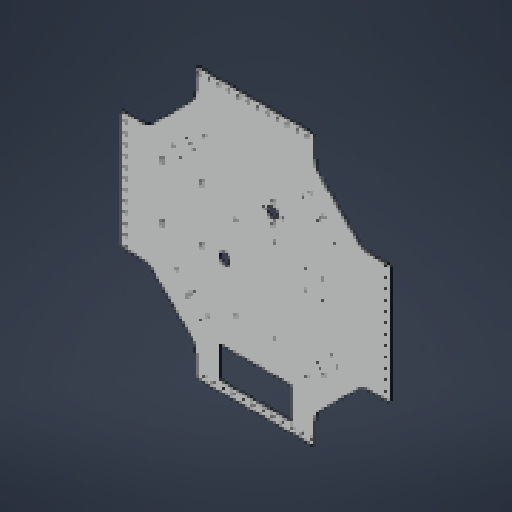
# Autodesk Inventor part: PLATE,MOUNT,ELECTRONICS
Saved by Autodesk Inventor 2026 (Build 300175000, 175)
## iProperties
Created: 2026-01-19
Part Number: PLATE,MOUNT,ELECTRONICS
Material: Aluminum 6061
Document SubType Name: Sheet Metal
Designer: Jthib
Mass: 2857.84 g
Surface Area: 7086.51 cm^2
Volume: 1058.46 cm^3
Density: 2.7 g/cm^3
Sheet Metal Rule: Default
Appearance: Aluminum - Flat
Flat Pattern Width: 69.85 cm
Flat Pattern Length: 69.85 cm
Flat Pattern Area: 4879.02 cm^2
Sheet Metal Width: 27.500 in
Sheet Metal Length: 27.500 in
Sheet Metal Area: 756.250 in^2
Author: Jthib
Autodesk Inventor part; units mm, degrees
ref_plane "YZ Plane" through (0, 0, 0) normal (1, 0, 0) x (0, 1, 0)
ref_plane "XZ Plane" through (0, 0, 0) normal (0, 1, 0) x (-1, 0, 0)
ref_plane "XY Plane" through (0, 0, 0) normal (0, 0, 1) x (1, 0, 0)
sketch "Sketch1" plane through (0, 0, 0) normal (0, 0, 1) x (1, 0, 0)
  line L0 (-298.45, -349.25) -> (298.45, -349.25)
  line L1 (349.25, -298.45) -> (349.25, 298.45)
  line L2 (298.45, 349.25) -> (-298.45, 349.25)
  line L3 (-349.25, 298.45) -> (-349.25, -298.45)
  line L4 (-349.25, -349.25) -> (349.25, 349.25) construction
  line L5 (349.25, -349.25) -> (-349.25, 349.25) construction
  arc A0 (349.25, 298.45) -> (298.45, 349.25) centre (298.45, 298.45) ccw
  arc A1 (-298.45, 349.25) -> (-349.25, 298.45) centre (-298.45, 298.45) ccw
  arc A2 (-349.25, -298.45) -> (-298.45, -349.25) centre (-298.45, -298.45) ccw
  arc A3 (298.45, -349.25) -> (349.25, -298.45) centre (298.45, -298.45) ccw
  point P0 (0, 0)
  dimension "d0" = 698.5
  dimension "d4" = 50.8
  measures "d0" distance of L4.end L5.end
  measures "d4" radius of A0
extrude "Plate1" add sketch "Sketch1" along normal blind 3.048
sketch "Sketch2" plane through (0, 0, 0) normal (0, 0, -1) x (-1, 0, 0)
  line L0 (-188.9125, -349.25) -> (-336.55, -349.25)
  arc A0 (-349.25, -336.55) -> (-336.55, -349.25) centre (-336.55, -336.55) ccw
  line L1 (-349.25, -336.55) -> (-349.25, -188.9125)
  line L2 (-153.035, -349.25) -> (-188.9125, -349.25)
  line L3 (-349.25, -188.9125) -> (-349.25, -153.035)
  line L4 (298.45, -349.25) -> (-298.45, -349.25) construction
  arc A1 (-270.7334, -168.4984) -> (-323.85, -190.5) centre (-292.735, -190.5) ccw construction
  line L5 (-270.7334, -168.4984) -> (-168.4984, -270.7334) construction
  arc A2 (-190.5, -323.85) -> (-168.4984, -270.7334) centre (-190.5, -292.735) ccw construction
  arc A3 (-266.2432, -164.0082) -> (-292.735, -153.035) centre (-292.735, -190.5) ccw
  line L6 (-266.2432, -164.0082) -> (-164.0082, -266.2432)
  arc A4 (-153.035, -292.735) -> (-164.0082, -266.2432) centre (-190.5, -292.735) ccw
  line L7 (-153.035, -349.25) -> (-153.035, -292.735)
  line L8 (-349.25, -153.035) -> (-292.735, -153.035)
  point P0 (0, 0)
  dimension "d10" = 6.35
  constraints: 16 end point, 10 point on circle, 5 centre point, 4 tangent, 2 perpendicular, 2 vertical, 1 collinear, 1 horizontal, 1 point on line, 15 other
  measures "d10" distance between parallel lines of L5 L6
extrude "Cut1" cut sketch "Sketch2" against normal blind 3.048
pattern_circular "Circular Pattern1" count 4 over 360 about axis through (0, 0, -10) along (0, 0, 1) of "Cut1"
fillet "Corner Round1" radius 6.35 8 edges at (-153.035, 349.25, 1.524) (349.25, -153.035, 1.524) (153.035, -349.25, 1.524) (-349.25, -153.035, 1.524) (-349.25, 153.035, 1.524) (-153.035, -349.25, 1.524) (153.035, 349.25, 1.524) (349.25, 153.035, 1.524)
sketch "Sketch3" plane through (0, 0, 0) normal (0, 0, -1) x (-1, 0, 0)
  line L0 (-146.685, 349.25) -> (146.685, 349.25) construction
  line L1 (-349.25, -146.685) -> (-349.25, 146.685) construction
  point P0 (0, 0)
  point P1 (-44.45, 120.65)
  point P2 (-19.05, 120.65)
  point P3 (-44.45, 146.05)
  point P4 (-69.85, 120.65)
  point P5 (-44.45, 95.25)
  dimension "d11" = 228.6
  dimension "d12" = 304.8
  dimension "d13" = 25.4
  dimension "d16" = 360
  constraints: 1 horizontal alignment, 5 other
  measures "d11" distance from line of L0 point (-44.45, 120.65)
  measures "d12" distance from line of L1 point (-44.45, 120.65)
  measures "d13" distance of point (-19.05, 120.65) point (-44.45, 120.65)
hole "Hole1" at (19.05, 120.65, 0) at (44.45, 146.05, 0) at (69.85, 120.65, 0) at (44.45, 95.25, 0) direction (0, 0, 1) diameter 5.1054 end through all clearance for "Flat Head Machine Screw (82)" size "#10" standard "Ansi Unified Screw Threads"
hole "Hole2" at (44.45, 120.65, 0) direction (0, 0, 1) diameter 28.575 end through all
sketch "Sketch4" plane through (0, 0, 3.048) normal (0, 0, 1) x (1, 0, 0)
  line L0 (-349.25, -146.685) -> (-349.25, 146.685) construction
  line L1 (-292.735, 153.035) -> (-342.9, 153.035) construction
  point P0 (0, 0)
  point P1 (-336.55, 133.35)
  dimension "d32" = 12.7
  dimension "d33" = 19.685
  measures "d32" distance from line of L0 point (-336.55, 133.35)
  measures "d33" distance from line of L1 point (-336.55, 133.35)
hole "Hole3" at (-336.55, 133.35, 3.048) direction (0, 0, -1) diameter 5.1054 end through all start extended yes clearance for "Flat Head Machine Screw (82)" size "#10" standard "Ansi Unified Screw Threads"
pattern_linear "Rectangular Pattern1" count 12 spacing 25.4 along (0, -1, 0) of "Hole3"
pattern_circular "Circular Pattern2" count 4 over 360 about axis through (0, 0, -10) along (0, 0, 1) of "Hole3", "Rectangular Pattern1"
sketch "Sketch5" plane through (0, 0, 3.048) normal (0, 0, 1) x (1, 0, 0)
  line L0 (-93.6625, -246.0625) -> (-93.6625, -320.675)
  line L1 (-90.4875, -323.85) -> (90.4875, -323.85)
  line L2 (93.6625, -320.675) -> (93.6625, -246.0625)
  line L3 (90.4875, -242.8875) -> (-90.4875, -242.8875)
  line L4 (-93.6625, -242.8875) -> (93.6625, -323.85) construction
  line L5 (-93.6625, -323.85) -> (93.6625, -242.8875) construction
  arc A0 (90.4875, -323.85) -> (93.6625, -320.675) centre (90.4875, -320.675) ccw
  arc A1 (-93.6625, -320.675) -> (-90.4875, -323.85) centre (-90.4875, -320.675) ccw
  arc A2 (-90.4875, -242.8875) -> (-93.6625, -246.0625) centre (-90.4875, -246.0625) ccw
  arc A3 (93.6625, -246.0625) -> (90.4875, -242.8875) centre (90.4875, -246.0625) ccw
  line L6 (146.685, -349.25) -> (-146.685, -349.25) construction
  line L7 (153.035, -342.9) -> (153.035, -292.735) construction
  line L8 (-153.035, -292.735) -> (-153.035, -342.9) construction
  point P0 (0, 0)
  point P1 (0, -283.3687)
  dimension "d47" = 80.9625
  dimension "d48" = 187.325
  dimension "d51" = 3.175
  dimension "d100" = 25.4
  dimension "d101" = 59.3725
  dimension "d102" = 59.3725
  constraints: 12 end point, 8 point on circle, 8 point on line, 8 tangent, 4 centre point, 3 equal radius, 2 midpoint, 2 parallel, 1 horizontal, 1 perpendicular
  measures "d47" distance of L4.end L5.end
  measures "d48" distance of L5.start L4.end
  measures "d51" radius of A0
  measures "d100" distance between parallel lines of L6 L1
  measures "d101" distance between parallel lines of L7 L2
  measures "d102" distance between parallel lines of L8 L0
extrude "Battery Cutout" cut sketch "Sketch5" against normal blind 3.048
sketch "Sketch6" plane through (0, 0, 0) normal (0, 0, -1) x (-1, 0, 0)
  circle A0 centre (-132.4208, -203.9623) radius 2.5 construction
  circle A1 centre (-177.322, -177.0215) radius 2.5 construction
  circle A2 centre (-168.0413, -168.3418) radius 2.5 construction
  circle A3 centre (-159.3615, -159.061) radius 2.5 construction
  circle A4 centre (-194.982, -123.4405) radius 2.5 construction
  circle A5 centre (-212.9426, -141.401) radius 2.5 construction
  point P0 (0, 0)
  constraints: 6 centre point, 12 other
hole "Hole4" at (132.4208, -203.9623, 0) at (177.322, -177.0215, 0) at (168.0413, -168.3418, 0) at (159.3615, -159.061, 0) at (194.982, -123.4405, 0) at (212.9426, -141.401, 0) direction (0, 0, 1) diameter 3.9624 end through all start extended yes thread size "10-32 UNF" class "2B" standard "ANSI Unified Screw Threads"
pattern_circular "Circular Pattern3" count 4 over 360 about axis through (0, 0, -10) along (0, 0, 1) of "Hole4"
sketch "Sketch7" plane through (0, 0, 0) normal (0, 0, -1) x (-1, 0, 0)
  line L0 (-50.8, -158.75) -> (-50.8, 57.15) construction
  line L1 (-50.8, 57.15) -> (50.8, 57.15) construction
  line L2 (50.8, 57.15) -> (50.8, -158.75) construction
  line L3 (50.8, -158.75) -> (-50.8, -158.75) construction
  line L4 (-50.8, -158.75) -> (50.8, 57.15) construction
  line L5 (-50.8, 57.15) -> (50.8, -158.75) construction
  line L6 (0, -488.95) -> (0, 488.95) construction
  line L7 (488.95, 0) -> (-488.95, 0) construction
  point P0 (0, 0)
  point P1 (0, -50.8)
  dimension "d65" = 215.9
  dimension "d66" = 101.6
  dimension "d87" = 0
  dimension "d103" = 50.8
  constraints: 12 end point, 3 midpoint, 2 parallel, 1 horizontal, 1 perpendicular
  measures "d65" distance of L1.end L2.end
  measures "d66" distance of L0.end L1.end
  measures "d87" distance from line of L6 point (0, -50.8)
  measures "d103" distance from line of L7 point (0, -50.8)
hole "Hole5" at (50.8, 57.15, 0) at (-50.8, 57.15, 0) at (-50.8, -158.75, 0) at (50.8, -158.75, 0) direction (0, 0, 1) diameter 3.9624 end through all start extended yes thread size "10-32 UNF" class "2B" standard "ANSI Unified Screw Threads"
sketch "Sketch8" plane through (0, 0, 0) normal (0, 0, -1) x (-1, 0, 0)
  line L0 (-130.8735, 36.576) -> (-130.8735, -11.176) construction
  line L1 (-130.8735, -11.176) -> (-173.9265, -11.176) construction
  line L2 (-173.9265, -11.176) -> (-173.9265, 36.576) construction
  line L3 (-173.9265, 36.576) -> (-130.8735, 36.576) construction
  line L4 (-130.8735, 36.576) -> (-173.9265, -11.176) construction
  line L5 (-130.8735, -11.176) -> (-173.9265, 36.576) construction
  line L6 (0, -488.95) -> (0, 488.95) construction
  line L7 (488.95, 0) -> (-488.95, 0) construction
  point P0 (0, 0)
  point P1 (-152.4, 12.7)
  dimension "d74" = 43.053
  dimension "d75" = 47.752
  dimension "d85" = 152.4
  dimension "d86" = 12.7
  constraints: 12 end point, 2 midpoint, 2 parallel, 1 horizontal, 1 perpendicular
  measures "d74" distance of L2.end L0.start
  measures "d75" distance of L1.end L2.end
  measures "d85" distance from line of point (-152.4, 12.7) L6
  measures "d86" distance from line of L7 point (-152.4, 12.7)
hole "Hole6" at (130.8735, -11.176, 0) at (173.9265, -11.176, 0) at (173.9265, 36.576, 0) at (130.8735, 36.576, 0) direction (0, 0, 1) diameter 3.302 end through all start extended yes thread size "8-32 UNC" class "2B" standard "ANSI Unified Screw Threads"
sketch "Sketch9" plane through (0, 0, 0) normal (0, 0, -1) x (-1, 0, 0)
  line L0 (139.7, -49.2125) -> (139.7, 100.0125) construction
  line L1 (139.7, 100.0125) -> (241.3, 100.0125) construction
  line L2 (241.3, 100.0125) -> (241.3, -49.2125) construction
  line L3 (241.3, -49.2125) -> (139.7, -49.2125) construction
  line L4 (139.7, -49.2125) -> (241.3, 100.0125) construction
  line L5 (139.7, 100.0125) -> (241.3, -49.2125) construction
  line L6 (241.3, 91.1225) -> (139.7, 91.1225) construction
  line L7 (139.7, -40.3225) -> (241.3, -40.3225) construction
  line L8 (0, -488.95) -> (0, 488.95) construction
  line L9 (-488.95, 0) -> (488.95, 0) construction
  point P0 (0, 0)
  point P1 (190.5, 25.4)
  dimension "d88" = 101.6
  dimension "d89" = 149.225
  dimension "d90" = 8.89
  dimension "d91" = 8.89
  dimension "d104" = 190.5
  dimension "d105" = 25.4
  constraints: 16 end point, 4 point on line, 3 perpendicular, 2 midpoint, 2 parallel, 1 vertical
  measures "d88" distance of L0.end L1.end
  measures "d89" distance of L0.start L0.end
  measures "d90" distance between parallel lines of L1 L6
  measures "d91" distance between parallel lines of L3 L7
  measures "d104" distance from line of point (190.5, 25.4) L8
  measures "d105" distance from line of L9 point (190.5, 25.4)
hole "Hole7" at (-139.7, 100.0125, 0) at (-139.7, 91.1225, 0) at (-139.7, -40.3225, 0) at (-139.7, -49.2125, 0) at (-241.3, -49.2125, 0) at (-241.3, -40.3225, 0) at (-241.3, 91.1225, 0) at (-241.3, 100.0125, 0) direction (0, 0, 1) diameter 5.1054 end through all start extended yes clearance for "Flat Head Machine Screw (82)" size "#10" standard "Ansi Unified Screw Threads"
sketch "Sketch11" plane through (0, 0, 3.048) normal (0, 0, 1) x (1, 0, 0)
  circle A0 centre (-76.962, -58.293) radius 14.2875
  line L0 (-285.75, -238.125) -> (349.25, -238.125) projected
  line L1 (-87.3496, -237.8) -> (-71.3496, -237.8) projected
  point P0 (0, 0)
  point P1 (-79.3496, -237.8)
  dimension "d113" = 28.575
  dimension "d114" = 179.832
  dimension "d120" = 208.788
  constraints: 1 centre point, 1 midpoint
  measures "d113" diameter of A0
  measures "d114" distance from line of L0 A0.centre
  measures "d120" horizontal distance of L0.start A0.centre
extrude "Cut3" cut sketch "Sketch11" against normal blind 3.048
equation "\"d2\" = Thickness"
equation "\"d23\" = Thickness"
equation "\"d39\" = Thickness"
equation "\"d101\" = d102"
equation "\"d52\" = Thickness"
equation "\"d90\" = d91"
equation "\"d117\" = Thickness"
equation "\"d1\" = Thickness"
equation "\"BendRadius\" = Thickness"
equation "\"BendReliefWidth\" = Thickness"
equation "\"BendReliefDepth\" = 0.5 * Thickness"
equation "\"CornerReliefSize\" = 4 * Thickness"
equation "\"MinimumRemnant\" = 2 * Thickness"
equation "\"TransitionRadius\" = BendRadius"
equation "\"JacobiRadiusSize\" = BendRadius"
equation "\"GapSize\" = Thickness"
equation "\"Thickness\" = 3.048"
body "Solid1"
